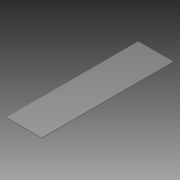
# Autodesk Inventor part: side
Saved by Autodesk Inventor 2014 SP1 (Build 180222100, 222)
## iProperties
Created: 2013-10-25
Part Number: side
Material: Polycarbonate, Clear
Document SubType Name: Modeling
Designer: RyanHughes
Density: 1.2 g/cm^3
Appearance: Polycarbonate - Clear
Author: RyanHughes
Autodesk Inventor part; units mm, degrees
ref_plane "YZ Plane" through (0, 0, 0) normal (1, 0, 0) x (0, 1, 0)
ref_plane "XZ Plane" through (0, 0, 0) normal (0, 1, 0) x (-1, 0, 0)
ref_plane "XY Plane" through (0, 0, 0) normal (0, 0, 1) x (1, 0, 0)
sketch "Sketch1" plane through (0, 0, 0) normal (0, 1, 0) x (-1, 0, 0)
  line L0 (25.4, -95.25) -> (-25.4, -95.25)
  line L1 (-25.4, -95.25) -> (-25.4, 95.25)
  line L2 (-25.4, 95.25) -> (25.4, 95.25)
  line L3 (25.4, 95.25) -> (25.4, -95.25)
  line L4 (25.4, -95.25) -> (-25.4, 95.25) construction
  line L5 (-25.4, -95.25) -> (25.4, 95.25) construction
  point P0 (0, 0)
  dimension "d0" = 50.8
  dimension "d1" = 190.5
  constraints: 12 end point, 2 midpoint, 2 parallel, 1 horizontal, 1 perpendicular
  measures "d0" distance of L1.end L2.end
  measures "d1" distance of L0.end L1.end
extrude "Extrusion1" add sketch "Sketch1" along normal blind 1.5875
body "Solid1"
